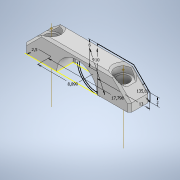
# Autodesk Inventor part: halter1_2
Saved by Autodesk Inventor 2022 (Build 260153000, 153)
## iProperties
Created: 2022-11-24
Part Number: halter1_2
Material: Generisch
Document SubType Name: Modeling
Designer: Friedrich Walmrath
Density: 1 g/cm^3
Appearance: Vorgabe
Author: Friedrich Walmrath
Autodesk Inventor part; units mm, degrees
ref_plane "YZ Plane" through (0, 0, 0) normal (1, 0, 0) x (0, 1, 0)
ref_plane "XZ Plane" through (0, 0, 0) normal (0, 1, 0) x (-1, 0, 0)
ref_plane "XY Plane" through (0, 0, 0) normal (0, 0, 1) x (1, 0, 0)
sketch "Skizze1" plane through (0, 0, 0) normal (0, 0, 1) x (1, 0, 0)
  circle A0 centre (0, 0) radius 4.5
  circle A1 centre (0, 0) radius 5
  line L0 (0, 0) -> (13, 0)
  line L1 (13, 0) -> (13, 2)
  line L2 (13, 2) -> (9, 6)
  line L3 (9, 6) -> (0, 6)
  line L4 (0, 6) -> (0, 0)
  point P0 (0, 4.5)
  point P1 (4.5, 0)
  point P2 (0, 5)
  point P3 (5, 0)
  dimension "d0" = 9
  dimension "d1" = 10
  dimension "d2" = 6
  dimension "d3" = 2
  dimension "d4" = 13
  dimension "d5" = 135
  constraints: 10 end point, 2 centre point, 2 coincident, 2 perpendicular, 1 horizontal, 1 parallel
  measures "d0" diameter of A0
  measures "d1" diameter of A1
  measures "d2" distance of L3.end L0.start
  measures "d3" distance of L0.end L1.end
  measures "d4" distance of L0.start L0.end
  measures "d5" angle of L1 L2
extrude "Extrusion1" add sketch "Skizze1" along normal blind 1 contours A0 L4 A1 L0 | A1 L4 L3 L2 L1 L0 picked at (4.7539, 0.7046)
extrude "Extrusion2" add sketch "Skizze1" along normal blind 5 contours A1 L4 L3 L2 L1 L0
mirror "Spiegeln1" about plane through (0, 6, 0) normal (-1, 0, 0)
sketch "Skizze2" plane through (4.5, 0, 0) normal (0, -1, 0) x (1, 0, 0)
  line L0 (-9.5, 1) -> (0.5, 1) projected
  line L1 (0.5, 1) -> (0.5, 5) projected
  line L2 (0.5, 5) -> (-9.5, 5) projected
  line L3 (-9.5, 1) -> (-9.5, 5) projected
  line L4 (-9.5, 1) -> (0.5, 1) projected
  line L5 (-9.5, 5) -> (-17.5, 5) projected
  point P0 (-4.5, 0)
  point P1 (-13.399, 2.5)
  point P2 (4.399, 2.5)
  point P3 (-4.5, 1)
  dimension "d10" = 17.798
  dimension "d11" = 8.899
  dimension "d12" = 2.5
  constraints: 2 midpoint, 1 horizontal alignment
  measures "d10" distance of point (4.399, 2.5) point (-13.399, 2.5)
  measures "d11" horizontal distance of point (-4.5, 1) point (-13.399, 2.5)
  measures "d12" distance from line of point (-13.399, 2.5) L5
hole "Bohrung2" at (-8.899, 6, 2.5) direction (0, -1, 0) diameter 3 end through all counterbore diameter 4 counterbore depth 2
hole "Bohrung3" at (8.899, 6, 2.5) direction (0, -1, 0) diameter 3 end through all counterbore diameter 4 counterbore depth 2
chamfer "Fase1" distance 0.5 angle 45 16 edges at (-10.899, 4.101, 2.5) (-6.8996, 6, 2.4495) (-8.9495, 6, 4.4994) (8.9495, 6, 4.4994) (6.8996, 6, 2.4495) (10.899, 4.101, 2.5) (0, 6, 5) (0, 6, 0) (-11, 4, 5) (-11, 4, 0) (11, 4, 5) (11, 4, 0) (-13, 1, 5) (-13, 1, 0) (13, 1, 5) (13, 1, 0)
